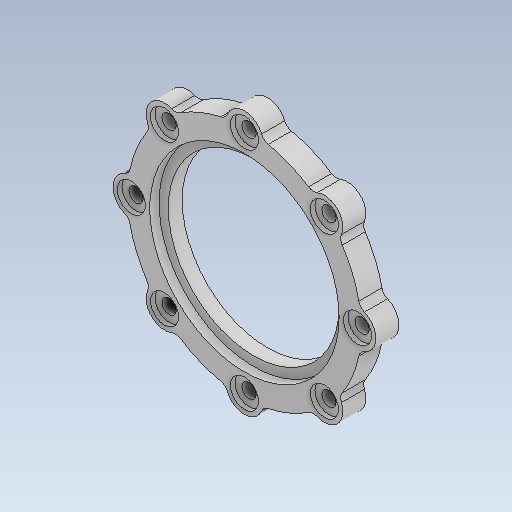
# Autodesk Inventor part: Outer_support_stand
Saved by Autodesk Inventor 2020.4 (Build 244396000, 396)
## iProperties
Created: 2021-09-25
Part Number: Outer_support_stand
Material: アルミニウム 2014-T4
Document SubType Name: Modeling
Designer: Masato Kubotera
Density: 2.8 g/cm^3
Appearance: 滑らか - 淡い灰色
Mass: 14.2998 g
Surface Area: 42.289 cm^2
Volume: 5.10707 cm^3
Author: Masato Kubotera
Autodesk Inventor part; units mm, degrees
ref_plane "YZ Plane" through (0, 0, 0) normal (1, 0, 0) x (0, 1, 0)
ref_plane "XZ Plane" through (0, 0, 0) normal (0, 1, 0) x (-1, 0, 0)
ref_plane "XY Plane" through (0, 0, 0) normal (0, 0, 1) x (1, 0, 0)
derived "Trunk_horizontal_frame_01.ipt"
sketch "スケッチ1" plane through (0, 0, 0) normal (0, 0, 1) x (1, 0, 0)
  line L0 (-62, 30.75) -> (62, 30.75)
  line L1 (62, -30.75) -> (-62, -30.75)
  line L2 (-62, 30.75) -> (62, -30.75) construction
  line L3 (62, 30.75) -> (-62, -30.75) construction
  line L4 (0, 30.75) -> (0, -30.75) construction
  circle A0 centre (-44, 2.25) radius 10.5 construction
  line L5 (-57.5, 1.25) -> (-30.5, 1.25) construction
  line L6 (-30.5, 1.25) -> (-30.5, -25.75) construction
  line L7 (-30.5, -25.75) -> (-57.5, -25.75) construction
  line L8 (-57.5, -25.75) -> (-57.5, 1.25) construction
  line L9 (-44, 1.25) -> (-44, -25.75) construction
  line L10 (-57.5, -12.25) -> (-30.5, -12.25) construction
  circle A1 centre (-57.5, 1.25) radius 1.35
  circle A2 centre (-57.5, -25.75) radius 1.35
  circle A3 centre (-30.5, 1.25) radius 1.35
  circle A4 centre (-30.5, -25.75) radius 1.35
  line L11 (-27.5, 21.75) -> (-22.5, 21.75) construction
  line L12 (-22.5, 21.75) -> (-22.5, 11.75) construction
  line L13 (-22.5, 11.75) -> (-27.5, 11.75) construction
  line L14 (-27.5, 11.75) -> (-27.5, 21.75) construction
  line L15 (-27.5, 21.75) -> (-22.5, 11.75) construction
  line L16 (-22.5, 21.75) -> (-27.5, 11.75) construction
  line L17 (-27.51, 21.76) -> (-22.49, 21.76)
  line L18 (-22.49, 21.76) -> (-22.49, 11.74)
  line L19 (-22.49, 11.74) -> (-27.51, 11.74)
  line L20 (-27.51, 11.74) -> (-27.51, 21.76)
  line L21 (-27.51, 21.76) -> (-22.49, 11.74) construction
  line L22 (-22.49, 21.76) -> (-27.51, 11.74) construction
  line L23 (-27.51, 16.75) -> (-22.49, 16.75) construction
  line L24 (-25, 21.76) -> (-25, 11.74) construction
  arc A5 (-27.51, 21.76) -> (-27.51, 19.66) centre (-27.51, 20.71) ccw
  arc A6 (-22.49, 19.66) -> (-22.49, 21.76) centre (-22.49, 20.71) ccw
  arc A7 (-22.49, 11.74) -> (-22.49, 13.84) centre (-22.49, 12.79) ccw
  arc A8 (-27.51, 13.84) -> (-27.51, 11.74) centre (-27.51, 12.79) ccw
  circle A9 centre (-25, 27.75) radius 1.55
  arc A10 (-27.51, -19.66) -> (-27.51, -21.76) centre (-27.51, -20.71) ccw
  line L25 (-22.5, -21.75) -> (-27.5, -21.75) construction
  line L26 (-22.49, -21.76) -> (-27.51, -21.76)
  arc A11 (-22.49, -21.76) -> (-22.49, -19.66) centre (-22.49, -20.71) ccw
  line L27 (-27.5, -21.75) -> (-27.5, -9.25) construction
  line L28 (-27.51, -21.76) -> (-27.51, -9.24)
  line L29 (-27.51, -15.5) -> (-22.49, -15.5) construction
  line L30 (-25, -9.24) -> (-25, -21.76) construction
  line L31 (-27.5, -9.25) -> (-22.5, -21.75) construction
  line L32 (-22.5, -9.25) -> (-27.5, -21.75) construction
  line L33 (-27.51, -9.24) -> (-22.49, -21.76) construction
  line L34 (-22.49, -9.24) -> (-27.51, -21.76) construction
  line L35 (-22.5, -9.25) -> (-22.5, -21.75) construction
  line L36 (-22.49, -9.24) -> (-22.49, -21.76)
  circle A12 centre (-25, -27.75) radius 1.55
  arc A13 (-22.49, -11.34) -> (-22.49, -9.24) centre (-22.49, -10.29) ccw
  line L37 (-27.5, -9.25) -> (-22.5, -9.25) construction
  line L38 (-27.51, -9.24) -> (-22.49, -9.24)
  arc A14 (-27.51, -9.24) -> (-27.51, -11.34) centre (-27.51, -10.29) ccw
  circle A15 centre (-44, 2.25) radius 11
  line L39 (62, 2.25) -> (-62, 2.25) construction
  line L40 (-60, 14.25) -> (-28, 14.25) construction
  line L41 (-28, 14.25) -> (-28, -28.75) construction
  line L42 (-28, -28.75) -> (-60, -28.75) construction
  line L43 (-60, -28.75) -> (-60, 14.25) construction
  line L44 (-60, 14.25) -> (-28, -28.75) construction
  line L45 (-28, 14.25) -> (-60, -28.75) construction
  line L46 (-62, 30.75) -> (-62, -30.75) construction
  line L47 (62, 30.75) -> (62, -30.75) construction
  circle A16 centre (-44, 2.25) radius 12.5 construction
  circle A17 centre (-44, 2.25) radius 20.5 construction
  circle A18 centre (-44, 2.25) radius 28.5 construction
  circle A19 centre (-44, 26.75) radius 2.2 construction
  circle A20 centre (-61.3241, 19.5741) radius 2.2 construction
  circle A21 centre (-68.5, 2.25) radius 2.2 construction
  circle A22 centre (-61.3241, -15.0741) radius 2.2 construction
  circle A23 centre (-44, -22.25) radius 2.2 construction
  circle A24 centre (-26.6759, -15.0741) radius 2.2 construction
  circle A25 centre (-19.5, 2.25) radius 2.2 construction
  circle A26 centre (-26.6759, 19.5741) radius 2.2 construction
  line L48 (-62, -21.122) -> (-62, -30.75)
  arc A27 (22.49, -9.24) -> (22.49, -11.34) centre (22.49, -10.29) ccw
  line L49 (27.51, -9.24) -> (22.49, -9.24)
  arc A28 (27.51, -11.34) -> (27.51, -9.24) centre (27.51, -10.29) ccw
  line L50 (27.51, -21.76) -> (27.51, -9.24)
  line L51 (22.49, -9.24) -> (22.49, -21.76)
  circle A29 centre (26.6759, -15.0741) radius 2.2
  arc A30 (27.51, -21.76) -> (27.51, -19.66) centre (27.51, -20.71) ccw
  line L52 (22.49, -21.76) -> (27.51, -21.76)
  arc A31 (22.49, -19.66) -> (22.49, -21.76) centre (22.49, -20.71) ccw
  circle A32 centre (25, -27.75) radius 1.55
  circle A33 centre (30.5, -25.75) radius 1.35
  circle A34 centre (44, -22.25) radius 2.2
  circle A35 centre (57.5, -25.75) radius 1.35
  circle A36 centre (61.3241, -15.0741) radius 2.2
  line L53 (62, -21.122) -> (62, -30.75)
  circle A37 centre (68.5, 2.25) radius 2.2
  circle A38 centre (61.3241, 19.5741) radius 2.2
  circle A39 centre (44, 26.75) radius 2.2
  circle A40 centre (44, 2.25) radius 11
  circle A41 centre (26.6759, 19.5741) radius 2.2
  circle A42 centre (25, 27.75) radius 1.55
  circle A43 centre (30.5, 1.25) radius 1.35
  circle A44 centre (57.5, 1.25) radius 1.35
  circle A45 centre (19.5, 2.25) radius 2.2
  line L54 (22.49, 11.74) -> (27.51, 11.74)
  arc A46 (27.51, 11.74) -> (27.51, 13.84) centre (27.51, 12.79) ccw
  arc A47 (22.49, 13.84) -> (22.49, 11.74) centre (22.49, 12.79) ccw
  line L55 (22.49, 21.76) -> (22.49, 11.74)
  line L56 (27.51, 11.74) -> (27.51, 21.76)
  arc A48 (22.49, 21.76) -> (22.49, 19.66) centre (22.49, 20.71) ccw
  line L57 (27.51, 21.76) -> (22.49, 21.76)
  arc A49 (27.51, 19.66) -> (27.51, 21.76) centre (27.51, 20.71) ccw
  circle A50 centre (-44, 2.25) radius 20.51
  circle A51 centre (-44, 2.25) radius 18.5
  circle A52 centre (-44, 2.25) radius 28.5
  circle A53 centre (-44, 26.75) radius 1.55
  circle A54 centre (-61.3241, 19.5741) radius 1.55
  circle A55 centre (-68.5, 2.25) radius 1.55
  circle A56 centre (-61.3241, -15.0741) radius 1.55
  circle A57 centre (-44, -22.25) radius 1.55
  circle A58 centre (-26.6759, -15.0741) radius 1.55
  circle A59 centre (-19.5, 2.25) radius 1.55
  circle A60 centre (-26.6759, 19.5741) radius 1.55
  line L58 (-68.5, 2.25) -> (-73.5, 2.25) construction
  circle A61 centre (-26.6759, 19.5741) radius 7.2 construction
  circle A62 centre (-19.5, 2.25) radius 7.2 construction
  circle A63 centre (-26.6759, -15.0741) radius 7.2 construction
  circle A64 centre (-44, 2.25) radius 24.5 construction
  circle A65 centre (-44, 26.75) radius 3.05
  circle A66 centre (-61.3241, 19.5741) radius 3.05
  circle A67 centre (-68.5, 2.25) radius 3.05
  circle A68 centre (-44, -22.25) radius 3.05
  circle A69 centre (-26.6759, -15.0741) radius 3.05
  circle A70 centre (-19.5, 2.25) radius 3.05
  circle A71 centre (-26.6759, 19.5741) radius 3.05
  circle A72 centre (-61.3241, -15.0741) radius 3.05
  circle A73 centre (-30.5, -25.75) radius 2.4
  arc A74 (-44, 30.75) -> (-47.969, 27.2469) centre (-44, 26.75) ccw
  arc A75 (-58.8689, 22.732) -> (-64.1525, 22.4025) centre (-61.3241, 19.5741) ccw
  arc A76 (-47.969, 27.2469) -> (-58.8689, 22.732) centre (-44, 2.25) ccw
  arc A77 (-64.1525, 22.4025) -> (-64.482, 17.1189) centre (-61.3241, 19.5741) ccw
  arc A78 (-64.482, 17.1189) -> (-68.9969, 6.219) centre (-44, 2.25) ccw
  arc A79 (-68.9969, 6.219) -> (-72.5, 2.25) centre (-68.5, 2.25) ccw
  arc A80 (-72.5, 2.25) -> (-68.9969, -1.719) centre (-68.5, 2.25) ccw
  arc A81 (-68.9969, -1.719) -> (-64.482, -12.6189) centre (-44, 2.25) ccw
  arc A82 (-64.482, -12.6189) -> (-64.1525, -17.9025) centre (-61.3241, -15.0741) ccw
  arc A83 (-64.1525, -17.9025) -> (-58.8689, -18.232) centre (-61.3241, -15.0741) ccw
  arc A84 (-58.8689, -18.232) -> (-47.969, -22.7469) centre (-44, 2.25) ccw
  arc A85 (-47.969, -22.7469) -> (-44, -26.25) centre (-44, -22.25) ccw
  arc A86 (-44, -26.25) -> (-40.031, -22.7469) centre (-44, -22.25) ccw
  arc A87 (-40.031, -22.7469) -> (-29.1311, -18.232) centre (-44, 2.25) ccw
  arc A88 (-29.1311, -18.232) -> (-23.8475, -17.9025) centre (-26.6759, -15.0741) ccw
  arc A89 (-23.8475, -17.9025) -> (-23.518, -12.6189) centre (-26.6759, -15.0741) ccw
  arc A90 (-23.518, -12.6189) -> (-19.0031, -1.719) centre (-44, 2.25) ccw
  arc A91 (-19.0031, -1.719) -> (-15.5, 2.25) centre (-19.5, 2.25) ccw
  arc A92 (-15.5, 2.25) -> (-19.0031, 6.219) centre (-19.5, 2.25) ccw
  arc A93 (-19.0031, 6.219) -> (-23.518, 17.1189) centre (-44, 2.25) ccw
  arc A94 (-23.518, 17.1189) -> (-23.8475, 22.4025) centre (-26.6759, 19.5741) ccw
  arc A95 (-23.8475, 22.4025) -> (-29.1311, 22.732) centre (-26.6759, 19.5741) ccw
  arc A96 (-29.1311, 22.732) -> (-40.031, 27.2469) centre (-44, 2.25) ccw
  arc A97 (-40.031, 27.2469) -> (-44, 30.75) centre (-44, 26.75) ccw
  arc A98 (-48.9902, 27.0632) -> (-58.017, 23.3242) centre (-44, 2.25) ccw
  arc A99 (-41, 30.75) -> (-48.9902, 27.0632) centre (-44, 26.75) ccw
  arc A100 (-58.017, 23.3242) -> (-65.0742, 16.267) centre (-61.3241, 19.5741) ccw
  arc A101 (-65.0742, 16.267) -> (-68.8132, 7.2402) centre (-44, 2.25) ccw
  arc A102 (-68.8132, 7.2402) -> (-68.8132, -2.7402) centre (-68.5, 2.25) ccw
  arc A103 (-68.8132, -2.7402) -> (-65.0742, -11.767) centre (-44, 2.25) ccw
  arc A104 (-65.0742, -11.767) -> (-62, -20.0282) centre (-61.3241, -15.0741) ccw
  line L59 (-62, -20.0282) -> (-62, -21.122)
  arc A105 (48.9902, 27.0632) -> (41, 30.75) centre (44, 26.75) ccw
  arc A106 (58.017, 23.3242) -> (48.9902, 27.0632) centre (44, 2.25) ccw
  arc A107 (65.0742, 16.267) -> (58.017, 23.3242) centre (61.3241, 19.5741) ccw
  arc A108 (68.8132, 7.2402) -> (65.0742, 16.267) centre (44, 2.25) ccw
  arc A109 (68.8132, -2.7402) -> (68.8132, 7.2402) centre (68.5, 2.25) ccw
  arc A110 (65.0742, -11.767) -> (68.8132, -2.7402) centre (44, 2.25) ccw
  arc A111 (62, -20.0282) -> (65.0742, -11.767) centre (61.3241, -15.0741) ccw
  line L60 (62, -20.0282) -> (62, -21.122)
  point P0 (0, 0)
  point P1 (-25, 16.75)
  point P2 (-25, -15.5)
  point P3 (-44, -7.25)
  point P4 (-23.326, 21.76)
  point P5 (-23.2248, 21.76)
  point P6 (-23.8475, 22.4025)
  point P7 (-44, 30.75)
  point P8 (-64.1525, -17.9025)
  point P9 (-44, -26.25)
  point P10 (-23.8475, -17.9025)
  point P11 (-15.5, 2.25)
  point P12 (-23.8475, 22.4025)
  dimension "d2" = 0.01
  dimension "d3" = 37
  dimension "d4" = 3.1
  dimension "d5" = 3.1
  dimension "d6" = 3.1
  dimension "d7" = 3.1
  dimension "d8" = 3.1
  dimension "d9" = 3.1
  dimension "d10" = 3.1
  dimension "d11" = 3.1
  dimension "d16" = 6.1
  dimension "d17" = 6.1
  dimension "d18" = 6.1
  dimension "d20" = 6.1
  dimension "d21" = 6.1
  dimension "d22" = 6.1
  dimension "d23" = 6.1
  dimension "d24" = 6.1
  dimension "d27" = 4.8
  dimension "d30" = 360
  measures "d2" radial gap between concentric circles of A17 A50
  measures "d3" diameter of A51
  measures "d4" diameter of A53
  measures "d5" diameter of A54
  measures "d6" diameter of A55
  measures "d7" diameter of A56
  measures "d8" diameter of A57
  measures "d9" diameter of A58
  measures "d10" diameter of A59
  measures "d11" diameter of A60
  measures "d16" diameter of A65
  measures "d17" diameter of A66
  measures "d18" diameter of A67
  measures "d20" diameter of A68
  measures "d21" diameter of A69
  measures "d22" diameter of A70
  measures "d23" diameter of A71
  measures "d24" diameter of A72
  measures "d27" radial gap between concentric circles of A50 A76
extrude "押し出し1" add sketch "スケッチ1" along normal blind 5 contours A97 A96 A95 A94 L17 A71 L20 A50 A14 L28 A69 A88 A87 A86 A85 A84 A83 A82 A81 A80 A79 A78 A77 A75 A76 A74 | A94 A93 L18 L19 A50 L20 A71 L17 | A93 A92 A91 A90 A13 L38 A50 L19 A7 L18 | A7 L18 | A50 L28 A14 | A88 L28 A69 A50 L38 L36 A90 A89 | A90 L36 A13 picked at (-27.7734, -10.754) picked at (-22.3943, -10.3142)
extrude "押し出し2" add sketch "スケッチ1" along normal blind 3 contours A50 L19 L20 | L20 A8 L19 A50 L38 A14 | L20 A8 | A14 L28 A50 | L38 A50 L28 picked at (-27.8728, -9.9602)
extrude "押し出し3" add sketch "スケッチ1" along normal blind 4 contours A71 L20 A60 L17 | L17 A5 A60 L20 A71 | L20 A60 A5 | A69 L28 A58 | L28 A58 A69 | A65 | A66 | A67 | A68 | A70 | A72 picked at (-27.8233, 21.0216)
fillet "フィレット1" radius 2 16 edges at (-40.031, -22.7469, 2.5) (-29.1311, -18.232, 2.5) (-23.518, -12.6189, 2.5) (-19.0031, -1.719, 2.5) (-19.0031, 6.219, 2.5) (-23.518, 17.1189, 2.5) (-29.1311, 22.732, 2.5) (-40.031, 27.2469, 2.5) (-58.8689, 22.732, 2.5) (-68.9969, 6.219, 2.5) (-47.969, 27.2469, 2.5) (-64.482, 17.1189, 2.5) (-68.9969, -1.719, 2.5) (-64.482, -12.6189, 2.5) (-47.969, -22.7469, 2.5) (-58.8689, -18.232, 2.5)
equation "\"d5\" = d4"
equation "\"d6\" = d4"
equation "\"d7\" = d4"
equation "\"d8\" = d4"
equation "\"d9\" = d4"
equation "\"d10\" = d4"
equation "\"d11\" = d4"
equation "\"d17\" = d16"
equation "\"d18\" = d16"
equation "\"d20\" = d16"
equation "\"d21\" = d16"
equation "\"d22\" = d16"
equation "\"d23\" = d16"
equation "\"d24\" = d16"
